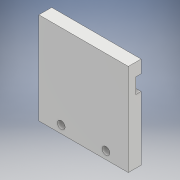
# Autodesk Inventor part: angle_clip
Saved by Autodesk Inventor 2017 (Build 210142000, 142)
## iProperties
Created: 2019-02-02
Part Number: angle_clip
Material: ABS Plastic
Document SubType Name: Modeling
Designer: simulator
Density: 1.06 g/cm^3
Appearance: Smooth - White
Mass: 2.44787 g
Surface Area: 18.1197 cm^2
Volume: 2.30931 cm^3
Author: simulator
## iProperties of the stored document angle_clip_3DPrint.ipt
Created: 2019-04-28
Part Number: angle_clip_3DPrint
Material: Generic
Document SubType Name: Modeling
Designer: simulator
Density: 1 g/cm^3
Appearance: Default
Author: simulator
Autodesk Inventor part; units mm, degrees
ref_plane "YZ Plane" through (0, 0, 0) normal (1, 0, 0) x (0, 1, 0)
ref_plane "XZ Plane" through (0, 0, 0) normal (0, 1, 0) x (-1, 0, 0)
ref_plane "XY Plane" through (0, 0, 0) normal (0, 0, 1) x (1, 0, 0)
sketch "Sketch1" plane through (0, 0, 0) normal (0, 1, 0) x (-1, 0, 0)
  line L0 (0, 0) -> (35, 0)
  line L1 (35, 0) -> (35, 6)
  line L2 (0, 6) -> (35, 6)
  line L3 (0, 0) -> (0, 6)
  line L4 (0, 6) -> (0, 0)
  line L5 (0, 3) -> (35, 3)
  line L6 (17.5, 3) -> (35, 3)
  line L7 (17.5, 3) -> (0, 3)
  point P0 (17.5, 0)
  point P1 (8.75, 3)
  point P2 (26.25, 3)
  constraints: 16 end point, 5 midpoint, 2 collinear
extrude "Extrusion1" add sketch "Sketch1" along normal blind 5
sketch "Sketch2" plane through (-35, 0, 6) normal (0, 0, 1) x (1, 0, 0)
  line L0 (0, 0) -> (35, 0) projected
  line L1 (35, 0) -> (35, 5) projected
  line L2 (0, 5) -> (35, 5) projected
  line L3 (0, 0) -> (0, 5) projected
extrude "Extrusion2" add sketch "Sketch2" along normal blind 30
sketch "Sketch3" plane through (0, 5, 0) normal (0, 1, 0) x (1, 0, 0)
  line L0 (0, 0) -> (0, -36) projected
  line L1 (0, 0) -> (-35, 0) projected
  line L2 (-35, 0) -> (-35, -36) projected
  line L3 (0, -36) -> (-35, -36) projected
  line L4 (-35, 0) -> (-35, -36) projected
  line L5 (-35, -31) -> (0, -31)
  line L6 (0, -31) -> (0, -25)
  line L7 (0, -25) -> (-35, -25)
  line L8 (-35, -25) -> (-35, -31)
  dimension "d4" = 5
  dimension "d5" = 25
  constraints: 8 end point, 2 parallel, 2 point on line, 1 horizontal, 1 perpendicular
  measures "d4" distance between parallel lines of L3 L5
  measures "d5" distance between parallel lines of L7 L1
extrude "Extrusion3" cut sketch "Sketch3" against normal blind 2 contours L0 L5 L2 L7
sketch "Sketch4" plane through (0, 0, 0) normal (0, -1, 0) x (1, 0, 0)
  line L0 (-35, 0) -> (0, 0)
  line L1 (0, 0) -> (0, 6)
  line L2 (-35, 6) -> (0, 6)
  line L3 (-35, 0) -> (-35, 6)
  line L4 (-35, 6) -> (-35, 0)
  line L5 (-35, 3) -> (0, 3)
  line L6 (-17.5, 3) -> (0, 3)
  line L7 (-17.5, 3) -> (-35, 3)
  point P0 (0, 0)
  point P1 (-17.5, 0)
  point P2 (-8.75, 3)
  point P3 (-26.25, 3)
  constraints: 16 end point, 5 midpoint, 2 collinear
hole "Hole1" at (-8.75, 0, 3) at (-26.25, 0, 3) direction (0, 1, 0) diameter 3 depth 8 tip angle 118
body "Solid1"
